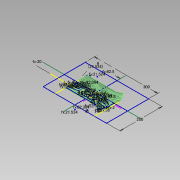
# Autodesk Inventor part: DoubleCross
Saved by Autodesk Inventor 2021 (Build 250183000, 183)
## iProperties
Created: 2021-02-18
Part Number: DoubleCross
Material: ABS プラスチック
Document SubType Name: Modeling
Designer: kumagai
Density: 1.06 g/cm^3
Appearance: 滑らか - 濃い深緑
Author: kumagai
Autodesk Inventor part; units mm, degrees
ref_plane "YZ Plane" through (0, 0, 0) normal (1, 0, 0) x (0, 1, 0)
ref_plane "XY Plane" through (0, 0, 0) normal (0, 0, 1) x (1, 0, 0)
sketch "スケッチ5" plane through (0, 0, 0) normal (0, 1, 0) x (-1, 0, 0)
  line L0 (0, -140) -> (0, 140) projected
  line L1 (-210, 0) -> (210, 0) projected
  line L2 (-150, 0) -> (-150, -100)
  line L3 (-150, -100) -> (0, -100)
  line L4 (0, -100) -> (0, 0)
  line L5 (150, 0) -> (150, -100)
  line L6 (150, -100) -> (0, -100)
  line L7 (0, -100) -> (0, 0)
  line L8 (150, 0) -> (150, 100)
  line L9 (150, 100) -> (0, 100)
  line L10 (0, 100) -> (0, 0)
  line L11 (0, 0) -> (-150, 0)
  line L12 (-150, 0) -> (-150, 100)
  line L13 (-150, 100) -> (0, 100)
  line L14 (0, 100) -> (0, 0)
  line L15 (150, 0) -> (0, 0)
  dimension "d218" = 300
  dimension "d219" = 200
  constraints: 28 end point, 4 collinear, 4 point on line, 1 horizontal, 2 other
  measures "d218" distance between parallel lines of L2 L5
  measures "d219" distance between parallel lines of L13 L3
sketch "スケッチ1" plane through (0, 0, 0) normal (0, 1, 0) x (-1, 0, 0)
  line L0 (0, -106.675) -> (0, 156.3939) projected
  line L1 (-148.4507, 0) -> (243.2043, 0) projected
  line L2 (92.5, -19.3127) -> (92.5, 102.6777)
  line L3 (187.2536, 30) -> (-35.7436, 30)
  line L4 (-47.1753, 49) -> (0, 49)
  line L5 (92.5, 49) -> (92.5, 11)
  line L6 (-17.8548, -8.3259) -> (39.6091, 18.47)
  line L7 (18.4304, 27.3517) -> (5.5723, 21.3558)
  line L8 (54.1505, 6.4934) -> (44.1126, 1.8126)
  arc A0 (83.5, 36.9) -> (44.0499, 28.1541) centre (83.5, -56.4468) ccw
  arc A1 (83.5, 39.3) -> (43.0357, 30.3293) centre (83.5, -56.4468) ccw
  line L9 (44.9578, 0) -> (40.2254, 0)
  line L10 (92.5, 11) -> (87.5, 11)
  line L11 (92.5, 13) -> (87.5, 13)
  line L12 (92.5, 36.9) -> (83.5, 36.9)
  line L13 (92.5, 39.3) -> (83.5, 39.3)
  line L14 (2.614, 23.1) -> (-2.614, 23.1)
  line L15 (2.614, 20.7) -> (-2.614, 20.7)
  line L16 (-1.944, 6.7068) -> (-12.3504, 1.8542)
  line L17 (-92.5, -19.3127) -> (-92.5, 102.6777)
  line L18 (22.026, 39.3) -> (-20.7601, 39.3)
  line L19 (18.479, 10.1405) -> (25.1011, 7.0526)
  line L20 (22.0057, 0) -> (10.5402, -5.3464)
  line L21 (26.5906, 13) -> (19.1129, 13)
  line L22 (16.3268, 0) -> (7.4183, -4.1541)
  line L23 (12.7183, 1.6826) -> (1.9241, 6.7161)
  arc A2 (27.5324, 23.1) -> (28.7324, 20.7) centre (28.7324, 22.2) ccw
  arc A3 (19.1129, 13) -> (18.479, 10.1405) centre (19.1129, 11.5) ccw
  line L24 (44.0499, 28.1541) -> (33.2113, 23.1)
  line L25 (43.0357, 30.3293) -> (27.5324, 23.1)
  line L26 (92.5, 47) -> (-47.1753, 47)
  arc A4 (2.614, 20.7) -> (5.5723, 21.3558) centre (2.614, 27.7) ccw
  arc A5 (2.614, 23.1) -> (4.558, 23.531) centre (2.614, 27.7) ccw
  arc A6 (27.376, 11.381) -> (26.5123, 8.1096) centre (30.7138, 8.75) ccw
  arc A7 (27.376, 11.381) -> (26.5906, 13) centre (26.5906, 12) ccw
  arc A8 (25.1011, 7.0526) -> (26.5123, 8.1096) centre (25.5237, 7.9589) ccw
  circle A9 centre (30.7138, 8.75) radius 1.05
  line L27 (81.4838, 23.2406) -> (80.3533, 26.9122)
  line L28 (78.4783, 27.9043) -> (55.4263, 20.8063)
  line L29 (83.5, 9) -> (83.5, 6.9715)
  line L30 (85.5, 9) -> (85.5, 7.1011)
  line L31 (44.9578, 0) -> (54.9958, 4.6808)
  line L32 (92.5, 20.7) -> (84.9244, 20.7)
  line L33 (54.72, 20.7) -> (28.7324, 20.7)
  line L34 (92.5, 23.1) -> (85.146, 23.1)
  line L35 (54.72, 23.1) -> (33.2113, 23.1)
  arc A10 (81.4838, 23.2406) -> (84.9244, 20.7) centre (84.9244, 24.3) ccw
  line L36 (83.7124, 24.1586) -> (82.5588, 27.9052)
  line L37 (78.0588, 30.2863) -> (54.72, 23.1)
  arc A11 (54.72, 20.7) -> (55.4263, 20.8063) centre (54.72, 23.1) ccw
  arc A12 (82.5588, 27.9052) -> (78.0588, 30.2863) centre (79.1182, 26.8458) ccw
  arc A13 (87.5, 11) -> (85.5, 9) centre (87.5, 9) ccw
  arc A14 (87.5, 13) -> (83.5, 9) centre (87.5, 9) ccw
  arc A15 (44.1126, 1.8126) -> (42.9578, 0) centre (44.9578, 0) ccw
  arc A16 (76.4374, 20.376) -> (50.8964, 13.4719) centre (83.5, -56.4468) ccw
  line L38 (50.8964, 13.4719) -> (43.8683, 10.1947)
  arc A17 (81.6181, 5.5209) -> (57.7899, 7.9492) centre (61.9765, -69.0938) ccw
  arc A18 (80.9893, 3.6182) -> (57.8984, 5.9522) centre (61.9765, -69.0938) ccw
  arc A19 (57.1393, 7.8025) -> (54.1505, 6.4934) centre (83.5, -56.4468) ccw
  arc A20 (57.8984, 5.9522) -> (54.9958, 4.6808) centre (83.5, -56.4468) ccw
  arc A21 (80.9893, 3.6182) -> (85.5, 7.1011) centre (81.9, 7.1011) ccw
  arc A22 (57.7899, 7.9492) -> (57.1393, 7.8025) centre (57.8984, 5.9522) ccw
  line L39 (19.2456, 27.8223) -> (30.3104, 35.57)
  line L40 (23.4236, 39.116) -> (29.9956, 37.355)
  line L41 (17.869, 29.7883) -> (26.4745, 35.8139)
  line L42 (17.4161, 29.5268) -> (4.558, 23.531)
  line L43 (26.4745, 35.8139) -> (22.8025, 36.7978)
  arc A23 (30.3104, 35.57) -> (29.9956, 37.355) centre (29.7368, 36.3891) ccw
  arc A24 (17.4161, 29.5268) -> (17.869, 29.7883) centre (16.1483, 32.2457) ccw
  arc A25 (22.8025, 36.7978) -> (22.026, 36.9) centre (22.026, 33.9) ccw
  arc A26 (23.4236, 39.116) -> (22.026, 39.3) centre (22.026, 33.9) ccw
  arc A27 (18.4304, 27.3517) -> (19.2456, 27.8223) centre (16.1483, 32.2457) ccw
  arc A28 (83.7124, 24.1586) -> (85.146, 23.1) centre (85.146, 24.6) ccw
  arc A29 (80.3533, 26.9122) -> (78.4783, 27.9043) centre (78.9197, 26.4708) ccw
  arc A30 (81.6181, 5.5209) -> (83.5, 6.9715) centre (82, 6.9715) ccw
  line L44 (17.8548, -8.3259) -> (-39.6091, 18.47)
  line L45 (-44.9578, 0) -> (-91.8632, 21.8723)
  line L46 (-44.1126, 1.8126) -> (-91.018, 23.685)
  line L47 (-91.8632, 21.8723) -> (-75.8037, 56.312)
  line L48 (-80.5134, 27.2826) -> (-87.7638, 30.6635)
  line L49 (-79.4991, 29.4577) -> (-86.7495, 32.8387)
  line L50 (-76.3325, 54.3519) -> (-76.649, 54.4994)
  arc A31 (-42.9578, 0) -> (-44.1126, 1.8126) centre (-44.9578, 0) ccw
  line L51 (-44.9578, 0) -> (-42.9578, 0)
  line L52 (-29.1517, 20.7) -> (-50.8213, 20.7)
  line L53 (-33.2113, 23.1) -> (-50.8213, 23.1)
  arc A32 (-79.4991, 29.4577) -> (-50.8213, 23.1) centre (-50.8213, 90.9575) ccw
  arc A33 (-80.5134, 27.2826) -> (-50.8213, 20.7) centre (-50.8213, 90.9575) ccw
  arc A34 (-29.1517, 20.7) -> (-28.5178, 23.5595) centre (-29.1517, 22.2) ccw
  line L54 (-27.3709, 10.6) -> (-23.1725, 10.6)
  line L55 (1.372, 2.9423) -> (-3.0209, -6.4784)
  line L56 (-33.0509, 7.9049) -> (-34.7643, 9.3426)
  line L57 (-27.8918, 10.5544) -> (-34.7643, 9.3426)
  line L58 (-28.3086, 12.918) -> (-38.1378, 11.1848)
  line L59 (-34.5936, 6.0664) -> (-38.6069, 9.434)
  line L60 (-19.1129, 13) -> (-27.3709, 13)
  arc A35 (-27.3709, 13) -> (-28.3086, 12.918) centre (-27.3709, 7.6) ccw
  line L61 (-2.9583, 8.8819) -> (-15.0104, 3.2619)
  arc A36 (-38.1378, 11.1848) -> (-38.6069, 9.434) centre (-37.9641, 10.2) ccw
  line L62 (3.4119, 8.6704) -> (14.4604, 3.5184)
  arc A37 (-27.3709, 10.6) -> (-27.8918, 10.5544) centre (-27.3709, 7.6) ccw
  line L63 (85.5, 7.1011) -> (85.5, 0)
  line L64 (-85.5, 0) -> (-85.5, 17.631)
  arc A38 (-85.5, 17.631) -> (-86.6548, 19.4436) centre (-87.5, 17.631) ccw
  line L65 (-19.876, 30.6739) -> (-4.558, 23.531)
  line L66 (22.026, 36.9) -> (-18.4957, 36.9)
  arc A39 (-19.876, 30.6739) -> (-18.4957, 36.9) centre (-24.8832, 35.05) ccw
  arc A40 (-22.97, 31.255) -> (-21.5454, 37.681) centre (-24.8832, 35.05) ccw
  line L67 (-22.9425, 29.4557) -> (-5.5723, 21.3558)
  arc A41 (-22.97, 31.255) -> (-22.9425, 29.4557) centre (-22.5199, 30.362) ccw
  arc A42 (-20.7601, 39.3) -> (-21.5454, 37.681) centre (-20.7601, 38.3) ccw
  arc A43 (-5.5723, 21.3558) -> (-2.614, 20.7) centre (-2.614, 27.7) ccw
  arc A44 (-4.558, 23.531) -> (-2.614, 23.1) centre (-2.614, 27.7) ccw
  circle A45 centre (-24.8832, 35.05) radius 1.05
  line L68 (-52.3756, 34.5673) -> (-76.2675, 37.8765)
  line L69 (-77.5476, 39.5681) -> (-76.9749, 43.7026)
  line L70 (-52.7048, 32.19) -> (-76.5968, 35.4991)
  line L71 (-28.5178, 23.5595) -> (-51.6905, 34.3651)
  line L72 (-78.7639, 46.9896) -> (-79.9031, 47.5209)
  line L73 (-33.2113, 23.1) -> (-52.7048, 32.19)
  line L74 (-79.7782, 44.8145) -> (-80.9174, 45.3457)
  line L75 (-79.9249, 39.8973) -> (-79.3522, 44.0318)
  arc A46 (-51.6905, 34.3651) -> (-52.3756, 34.5673) centre (-52.7048, 32.19) ccw
  arc A47 (-79.3522, 44.0318) -> (-79.7782, 44.8145) centre (-80.0951, 44.1347) ccw
  arc A48 (-77.5476, 39.5681) -> (-76.2675, 37.8765) centre (-76.0618, 39.3623) ccw
  arc A49 (-79.9249, 39.8973) -> (-76.5968, 35.4991) centre (-76.0618, 39.3623) ccw
  arc A50 (-76.9749, 43.7026) -> (-78.7639, 46.9896) centre (-80.0951, 44.1347) ccw
  line L76 (-73.6747, 55.3192) -> (-71.9721, 58.9703)
  line L77 (-75.4873, 56.1645) -> (-73.7848, 59.8155)
  line L78 (-75.4873, 56.1645) -> (-75.8037, 56.312)
  arc A51 (-69.6536, 59.4897) -> (-71.9721, 58.9703) centre (-70.6127, 58.3364) ccw
  arc A52 (-68.3747, 61.0274) -> (-49.0894, 49.3809) centre (-20.3186, 118.8126) ccw
  arc A53 (-49.0894, 49.3809) -> (-47.1753, 49) centre (-47.1753, 54) ccw
  arc A54 (-69.6536, 59.4897) -> (-49.855, 47.5332) centre (-20.3186, 118.8126) ccw
  arc A55 (-49.855, 47.5332) -> (-47.1753, 47) centre (-47.1753, 54) ccw
  arc A56 (-68.3747, 61.0274) -> (-73.7848, 59.8155) centre (-70.6127, 58.3364) ccw
  arc A57 (-76.3325, 54.3519) -> (-73.6747, 55.3192) centre (-75.4873, 56.1645) ccw
  line L79 (0, 49) -> (92.5, 49)
  arc A58 (0.7304, 8.9235) -> (0, 9.1133) centre (0, 7.6133) ccw
  line L80 (16.4242, 0.1747) -> (0.7304, 8.9235)
  arc A59 (16.1268, 0) -> (16.4242, 0.1747) centre (16.3268, 0) ccw
  line L81 (17.5928, 2.271) -> (1.899, 11.0198)
  arc A60 (18.9268, 0) -> (17.5928, 2.271) centre (16.3268, 0) ccw
  arc A61 (1.899, 11.0198) -> (0, 11.5133) centre (0, 7.6133) ccw
  line L82 (18.9268, 0) -> (16.1268, 0)
  line L83 (0, 9.1133) -> (0, 11.5133)
  line L84 (-18.479, 10.1405) -> (-28.8404, 5.3089)
  line L85 (-0.7304, 8.9235) -> (-16.4242, 0.1747)
  line L86 (-1.899, 11.0198) -> (-17.5928, 2.271)
  arc A62 (0, 9.1133) -> (-0.7304, 8.9235) centre (0, 7.6133) ccw
  arc A63 (0, 11.5133) -> (-1.899, 11.0198) centre (0, 7.6133) ccw
  arc A64 (-16.4242, 0.1747) -> (-16.5268, 0) centre (-16.3268, 0) ccw
  arc A65 (-17.5928, 2.271) -> (-18.9268, 0) centre (-16.3268, 0) ccw
  line L87 (-16.5268, 0) -> (-18.9268, 0)
  line L88 (-23.1725, 10.6) -> (-29.8547, 7.4841)
  line L89 (-3.2266, -8.7568) -> (-12.1876, -4.5782)
  line L90 (-1.8881, -6.7329) -> (-16.3268, 0)
  arc A66 (-34.5936, 6.0664) -> (-28.8404, 5.3089) centre (-31.1225, 10.203) ccw
  arc A67 (-18.479, 10.1405) -> (-19.1129, 13) centre (-19.1129, 11.5) ccw
  arc A68 (-33.0509, 7.9049) -> (-29.8547, 7.4841) centre (-31.1225, 10.203) ccw
  point P0 (0, 0)
  point P1 (-4.1659, 20.7)
  point P2 (-3.6338, 23.1)
  point P3 (-24.8832, 39.3)
  point P4 (4.1659, 20.7)
  point P5 (3.6338, 23.1)
  point P6 (83.5, 13)
  point P7 (85.5, 11)
  point P8 (82.2661, 20.7)
  point P9 (79.9119, 28.3458)
  point P10 (83.5, 5)
  point P11 (84.0383, 23.1)
  point P12 (82.4959, 5.2843)
  point P13 (0, 39.3)
  point P14 (0, 23.1)
  point P15 (0, 20.7)
  point P16 (0, 47)
  point P17 (0, 49)
  point P18 (42.9578, 0)
  point P19 (-16.3268, 0)
  point P20 (32.0671, 36.8)
  point P21 (-48.5339, 47)
  point P22 (-40.2497, 10.8124)
  point P23 (-31.5868, 6.6764)
  point P24 (-17.4937, 10.6)
  point P25 (-26.6793, 31.1982)
  point P26 (-76.6558, 46.0066)
  point P27 (0, 36.9)
  point P28 (-71.139, 60.7571)
  point P29 (-71.8049, 64.0614)
  point P30 (-48.1525, 49)
  point P31 (16.5268, 0)
  dimension "d0" = 92.5
  dimension "d1" = 30
  dimension "d6" = 25
  dimension "d14" = 18.6
  dimension "d15" = 2.4
  dimension "d16" = 38
  dimension "d25" = 1.5
  dimension "d27" = 9
  dimension "d29" = 1.5
  dimension "d30" = 2
  dimension "d31" = 2
  dimension "d32" = 34
  dimension "d36" = 7
  dimension "d38" = 8.5
  dimension "d41" = 1
  dimension "d42" = 1
  dimension "d43" = 2.1
  dimension "d44" = 8
  dimension "d45" = 2
  dimension "d50" = 52.7863
  dimension "d51" = 52.7863
  dimension "d54" = 2.4
  dimension "d55" = 2.4
  dimension "d58" = 2
  dimension "d67" = 82.0938
  dimension "d68" = 21.5235
  dimension "d69" = 8
  dimension "d70" = 21.5235
  dimension "d73" = 2
  dimension "d74" = 82.0938
  dimension "d85" = 77.1468
  dimension "d91" = 2.4
  dimension "d94" = 1
  dimension "d95" = 3
  dimension "d103" = 1.5
  dimension "d104" = 3.6
  dimension "d105" = 2
  dimension "d110" = 92.5
  dimension "d117" = 8
  dimension "d118" = 8
  dimension "d120" = 1.5
  dimension "d123" = 10
  dimension "d125" = 15
  dimension "d126" = 2.5
  dimension "d127" = 2.4
  dimension "d128" = 10
  dimension "d131" = 18.6
  dimension "d132" = 2.4
  dimension "d140" = 1
  dimension "d150" = 2.4
  dimension "d151" = 3
  dimension "d152" = 2
  dimension "d154" = 8.5
  dimension "d155" = 1
  dimension "d159" = 2.4
  dimension "d160" = 2.1
  dimension "d161" = 52.7863
  dimension "d162" = 8
  dimension "d164" = 0.75
  dimension "d165" = 1.5
  dimension "d171" = 2.8
  dimension "d172" = 2.8
  dimension "d175" = 21.5235
  dimension "d177" = 8
  constraints: 180 end point, 145 point on circle, 109 tangent, 69 centre point, 59 point on line, 26 coincident, 22 collinear, 22 parallel, 14 perpendicular, 9 symmetric about line, 6 equal radius, 5 horizontal, 5 vertical, 1 vertical alignment, 31 other
  measures "d0" distance between parallel lines of L0 L2
  measures "d1" distance of the line from the sketch origin of L3
  measures "d6" angle to the sketch x axis of L6
  measures "d14" distance of L13.start L32.start
  measures "d15" distance of L32.start L34.start
  measures "d16" distance of L5.start L5.end
  measures "d25" radius of A3
  measures "d27" distance from line of A0.centre L2
  measures "d29" radius of A2
  measures "d30" distance between parallel lines of L4 L26
  measures "d31" distance of L5.end L11.start
  measures "d32" distance between parallel lines of L7 L8
  measures "d36" radius of A4
  measures "d38" diameter of A6
  measures "d41" radius of A7
  measures "d42" radius of A8
  measures "d43" diameter of A9
  measures "d44" distance of point (79.912, 28.346) point (82.266, 20.7)
  measures "d45" distance between parallel lines of L29 L30
  measures "d50" distance from line of L29 A6.centre
  measures "d51" distance from line of L27 A6.centre
  measures "d54" distance between parallel lines of L27 L36
  measures "d55" distance between parallel lines of L28 L37
  measures "d58" radius of A13
  measures "d67" distance from line of L28 A0.centre
  measures "d68" distance from line of L27 A0.centre
  measures "d69" vertical distance of L11.start point (83.5, 5)
  measures "d70" horizontal distance of A17.centre point (83.5, 5)
  measures "d73" radial gap between concentric circles of A17 A18
  measures "d74" vertical distance of A17.centre L11.start
  measures "d85" radius of A16
  measures "d91" distance between parallel lines of L42 L7
  measures "d94" radius of A23
  measures "d95" radius of A24
  measures "d103" radius of A28
  measures "d104" radius of A10
  measures "d105" distance between parallel lines of L8 L31
  measures "d110" distance from line of point (0, 0) L47
  measures "d117" distance from line of L47 A33.centre
  measures "d118" distance from line of L47 A32.centre
  measures "d120" radius of A34
  measures "d123" angle of L39 L7
  measures "d125" angle of L40 L18
  measures "d126" distance from line of point (32.067, 36.8) L18
  measures "d127" distance between parallel lines of L60 L54
  measures "d128" angle of L58 L60
  measures "d131" distance between parallel lines of L61 L20
  measures "d132" distance between parallel lines of L20 L22
  measures "d140" radius of A36
  measures "d150" distance between parallel lines of L58 L57
  measures "d151" radius of A37
  measures "d152" radius of A38
  measures "d154" diameter of A40
  measures "d155" radius of A41
  measures "d159" radial gap between concentric circles of A39 A40
  measures "d160" diameter of A45
  measures "d161" distance from line of A40.centre L69
  measures "d162" distance from line of point (-76.656, 46.007) L68
  measures "d164" radius of A47
  measures "d165" radius of A48
  measures "d171" distance from line of point (32.067, 36.8) L7
  measures "d172" distance from line of A36.centre L60
  measures "d175" distance from line of A54.centre L76
  measures "d177" distance from line of point (-71.139, 60.757) L50
sketch "スケッチ4" plane through (0, 0, 0) normal (0, 1, 0) x (-1, 0, 0)
  line L0 (85.5, 7.1011) -> (85.5, 0) projected
  line L1 (85.5, 9) -> (85.5, 7.1011) projected
  arc A0 (87.5, 11) -> (85.5, 9) centre (87.5, 9) ccw projected
  line L2 (92.5, 11) -> (87.5, 11) projected
  line L3 (92.5, 49) -> (92.5, 11) projected
  line L4 (0, 0) -> (85.5, 0)
  circle A1 centre (30.7138, 8.75) radius 1.05 projected
  circle A2 centre (-24.8832, 35.05) radius 1.05 projected
  line L5 (-85.5, 0) -> (-85.5, 17.631) projected
  arc A3 (-85.5, 17.631) -> (-86.6548, 19.4436) centre (-87.5, 17.631) ccw projected
  arc A4 (-49.0894, 49.3809) -> (-47.1753, 49) centre (-47.1753, 54) ccw projected
  arc A5 (-68.3747, 61.0274) -> (-49.0894, 49.3809) centre (-20.3186, 118.8126) ccw projected
  arc A6 (-68.3747, 61.0274) -> (-73.7848, 59.8155) centre (-70.6127, 58.3364) ccw projected
  line L6 (-75.4873, 56.1645) -> (-73.7848, 59.8155) projected
  line L7 (-75.4873, 56.1645) -> (-75.8037, 56.312) projected
  line L8 (-91.8632, 21.8723) -> (-75.8037, 56.312) projected
  line L9 (-86.6548, 19.4436) -> (-91.8632, 21.8723)
  line L10 (0, 0) -> (-85.5, 0)
  line L11 (0, 49) -> (92.5, 49) projected
  line L12 (-47.1753, 49) -> (0, 49) projected
  line L13 (0, 49) -> (0, 0)
  constraints: 8 end point
ref_plane "作業平面1" through (0, -5.2, 0) normal (0, 1, 0) x (-1, 0, 0)
sketch "スケッチ3" plane through (0, -5.2, 0) normal (0, 1, 0) x (-1, 0, 0)
  line L0 (0, 61.0234) -> (0, -23.1406) projected
  line L1 (-117.5528, 0) -> (57.8165, 0) projected
  line L2 (-26.9332, 33.8664) -> (-26.9332, 36.2336)
  line L3 (-26.9332, 36.2336) -> (-24.8832, 37.4171)
  line L4 (-24.8832, 37.4171) -> (-22.8332, 36.2336)
  line L5 (-22.8332, 36.2336) -> (-22.8332, 33.8664)
  line L6 (-22.8332, 33.8664) -> (-24.8832, 32.6829)
  line L7 (-24.8832, 32.6829) -> (-26.9332, 33.8664)
  line L8 (30.7138, 6.3829) -> (28.6638, 7.5664)
  line L9 (28.6638, 7.5664) -> (28.6638, 9.9336)
  line L10 (28.6638, 9.9336) -> (30.7138, 11.1171)
  line L11 (30.7138, 11.1171) -> (32.7638, 9.9336)
  line L12 (32.7638, 9.9336) -> (32.7638, 7.5664)
  line L13 (32.7638, 7.5664) -> (30.7138, 6.3829)
  point P0 (0, 0)
  point P1 (-24.8832, 35.05)
  point P2 (-24.8832, 35.05)
  point P3 (30.7138, 8.75)
  point P4 (30.7138, 8.75)
  dimension "d200" = 4.1
  dimension "d201" = 4.1
  constraints: 24 end point, 2 coincident, 2 vertical, 26 other
  measures "d200" distance between parallel lines of L5 L2
  measures "d201" distance between parallel lines of L12 L9
extrude "ST_R" add sketch "スケッチ1" along normal blind 3.2 contours L0 A61 L81 L6 L80 A58 | L19 A3 L21 A7 L6 | L6 A7 A6 A8 L19 | L0 L14 A5 L42 A24 L41 L3 L39 A27 L7 A4 L15 | L6 L81 A60 L1 A59 L80 | L0 L18 A26 L40 A23 L39 L3 L41 L43 A25 L66 | A15 L8 A19 A22 A17 A30 L29 A14 L11 L2 L10 A13 L30 A21 A18 A20 L31 L1 | L0 L79 L2 L26 | L25 A1 L13 L2 L12 A0 L3 | L3 A0 L24 L35 L37 A12 L36 A28 L34 L2 L32 A10 L27 A29 L28 A11 L33 A2 L25 | L37 A12 L3
extrude "ST_B" add sketch "スケッチ4" against normal blind 5.2 contours L0 L4 L13 L11 L3 L2 A0 L1
extrude "ST_H" cut sketch "スケッチ3" along normal blind 2.5 contours L8 L9 L10 L11 L12 L13
extrude "SL_R" add sketch "スケッチ1" along normal blind 3.2 contours A62 L85 L44 L86 A63 L0 | L84 A66 L59 A36 L58 A35 L44 | L44 A35 L60 A67 L84 | L15 A43 L67 A41 L3 L65 A44 L14 L0 | L85 A64 L1 A65 L86 L44 | L66 A39 L65 L3 A41 A40 A42 L18 L0 | L1 L45 L47 L46 A31 | L26 A55 A54 A51 L76 A57 L50 L47 L78 L77 A56 A52 A53 L4 L0 | L47 L49 A32 L53 L73 L70 A49 L75 A47 L74 L72 A50 L69 A48 L68 A46 L71 A34 L52 A33 L48
extrude "SL_B" add sketch "スケッチ4" against normal blind 5.2 contours L10 L5 A3 L9 L8 L7 L6 A6 A5 A4 L12 L13
extrude "SL_H" cut sketch "スケッチ3" along normal blind 2.5 contours L2 L3 L4 L5 L6 L7
mirror "ミラー3" about plane through (0, 0, 0) normal (0, 0, 1) of "ST_R", "ST_B", "ST_H", "SL_R", "SL_B", "SL_H"
extrude "M_ST_R" [suppressed]
extrude "M_ST_M" [suppressed]
extrude "M_SL_R" [suppressed]
extrude "M_SL_M" [suppressed]
